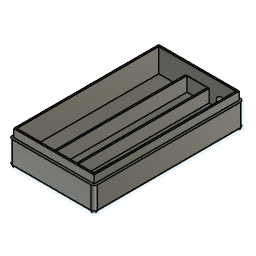
Controller_Left_Top v7 (Autodesk Fusion 360 design; units mm, degrees)
Autodesk Fusion 360 part; units mm, degrees
sketch "Sketch1" plane through (0, 0, 0) normal (0, 0, 1) x (1, 0, 0)
  line L0 (-27, -47.5) -> (27, -47.5)
  line L1 (27, -47.5) -> (27, 47.5)
  line L2 (27, 47.5) -> (-27, 47.5)
  line L3 (-27, 47.5) -> (-27, -47.5)
  line L4 (-27, -47.5) -> (27, 47.5) construction
  line L5 (27, -47.5) -> (-27, 47.5) construction
  dimension "d1" = 95
  dimension "d2" = 54
  constraint horizontal L0
  constraint perpendicular L0 L1
  constraint parallel L0 L2
  constraint parallel L1 L3
  constraint coincident L4 origin
  constraint coincident L5 origin
  measures "d1" distance of L0 L2
  measures "d2" distance of L1 L3
extrude "Extrude1" add sketch "Sketch1" along normal blind 11
sketch "Sketch2" plane through (0, 0, 11) normal (0, 0, 1) x (-1, 0, 0)
  line L0 (27, -47.5) -> (27, 47.5)
  line L1 (27, 47.5) -> (-27, 47.5)
  line L2 (-27, 47.5) -> (-27, -47.5)
  line L3 (-27, -47.5) -> (27, -47.5)
  line L4 (24.5, -45) -> (-24.5, -45)
  line L5 (-24.5, -45) -> (-24.5, 45)
  line L6 (-24.5, 45) -> (24.5, 45)
  line L7 (24.5, 45) -> (24.5, -45)
  line L8 (24.5, -45) -> (-24.5, 45) construction
  line L9 (-24.5, -45) -> (24.5, 45) construction
  dimension "d5" = 2.5
  dimension "d6" = 2.5
  dimension "d7" = 2.5
  dimension "d8" = 90
  constraint horizontal L4
  constraint perpendicular L4 L5
  constraint parallel L4 L6
  constraint parallel L5 L7
  constraint coincident L8 origin
  constraint coincident L9 origin
  measures "d5" distance of L3 L4
  measures "d6" distance of L1 L6
  measures "d7" distance of L2 L5
  measures "d8" distance of L4 L6
extrude "Extrude2" add sketch "Sketch2" along normal blind 5
extrude "Extrude3" cut 1 faces at (-8.1667, -15, 11) along direction (0, 0, -1) blind 5
sketch "Sketch3" plane through (0, 0, 6) normal (0, 0, 1) x (-1, 0, 0)
  line L0 (-24.5, 45) -> (-24.5, -45)
  line L1 (-24.5, -45) -> (24.5, -45)
  line L2 (24.5, -45) -> (24.5, 45)
  line L3 (24.5, 45) -> (-24.5, 45)
  line L4 (7.5, 45) -> (-7.5, 45)
  line L5 (-7.5, 45) -> (-7.5, -45)
  line L6 (-7.5, -45) -> (7.5, -45)
  line L7 (7.5, -45) -> (7.5, 45)
  line L8 (7.5, 45) -> (-7.5, -45) construction
  line L9 (-7.5, 45) -> (7.5, -45) construction
  dimension "d13" = 90
  dimension "d14" = 15
  constraint horizontal L4
  constraint perpendicular L4 L5
  constraint parallel L4 L6
  constraint parallel L5 L7
  constraint coincident L8 origin
  constraint coincident L9 origin
  measures "d13" distance of L4 L6
  measures "d14" distance of L5 L7
extrude "Extrude4" add sketch "Sketch3" along normal blind 8 contours L1 L3 L4 L5 L6 L7
sketch "Sketch4" plane through (0, 0, 14) normal (0, 0, 1) x (-1, 0, 0)
  line L0 (7.5, -45) -> (7.5, 45)
  line L1 (7.5, 45) -> (-7.5, 45)
  line L2 (-7.5, 45) -> (-7.5, -45)
  line L3 (-7.5, -45) -> (7.5, -45)
  line L4 (-6.5, 44.9) -> (6.5, 44.9)
  line L5 (6.5, 44.9) -> (6.5, -44.9)
  line L6 (6.5, -44.9) -> (-6.5, -44.9)
  line L7 (-6.5, -44.9) -> (-6.5, 44.9)
  line L8 (-6.5, 44.9) -> (6.5, -44.9) construction
  line L9 (6.5, 44.9) -> (-6.5, -44.9) construction
  dimension "d18" = 0.1
  dimension "d68" = 13
  constraint horizontal L4
  constraint perpendicular L4 L5
  constraint parallel L4 L6
  constraint parallel L5 L7
  constraint coincident L8 origin
  constraint coincident L9 origin
  measures "d18" distance of L3 L6
  measures "d68" distance of L5 L7
extrude "Extrude5" cut sketch "Sketch4" against normal blind 9 contours L4 L5 L6 L7
sketch "Sketch5" plane through (0, 0, 5) normal (0, 0, 1) x (-1, 0, 0)
  line L0 (-6.5, -44.9) -> (6.5, -44.9)
  line L1 (6.5, -44.9) -> (6.5, 44.9)
  line L2 (6.5, 44.9) -> (-6.5, 44.9)
  line L3 (-6.5, 44.9) -> (-6.5, -44.9)
  line L4 (-1.5, 36.5) -> (1.5, 36.5)
  line L5 (1.5, 36.5) -> (1.5, -36.5)
  line L6 (1.5, -36.5) -> (-1.5, -36.5)
  line L7 (-1.5, -36.5) -> (-1.5, 36.5)
  line L8 (-1.5, 36.5) -> (1.5, -36.5) construction
  line L9 (1.5, 36.5) -> (-1.5, -36.5) construction
  dimension "d21" = 3
  dimension "d22" = 73
  constraint horizontal L4
  constraint perpendicular L4 L5
  constraint parallel L4 L6
  constraint parallel L5 L7
  constraint coincident L8 origin
  constraint coincident L9 origin
  measures "d21" horizontal distance of L4.start L5.end
  measures "d22" distance of L4 L6
extrude "Extrude6" cut sketch "Sketch5" against normal blind 5 contours L4 L5 L6 L7
sketch "Sketch6" plane through (0, 0, 16) normal (0, 0, 1) x (-1, 0, 0)
  line L0 (-24.5, 45) -> (24.5, 45)
  line L1 (24.5, 45) -> (24.5, -45)
  line L2 (24.5, -45) -> (-24.5, -45)
  line L3 (-24.5, -45) -> (-24.5, 45)
  line L4 (-27, -47.5) -> (27, -47.5)
  line L5 (27, -47.5) -> (27, 47.5)
  line L6 (27, 47.5) -> (-27, 47.5)
  line L7 (-27, 47.5) -> (-27, -47.5)
  line L8 (-25.5, -46) -> (25.5, -46)
  line L9 (25.5, -46) -> (25.5, 46)
  line L10 (25.5, 46) -> (-25.5, 46)
  line L11 (-25.5, 46) -> (-25.5, -46)
  line L12 (-25.5, -46) -> (25.5, 46) construction
  line L13 (25.5, -46) -> (-25.5, 46) construction
  dimension "d25" = 1.5
  dimension "d26" = 1.5
  constraint horizontal L8
  constraint perpendicular L8 L9
  constraint parallel L8 L10
  constraint parallel L9 L11
  constraint coincident L12 origin
  constraint coincident L13 origin
  measures "d25" distance of L5 L9
  measures "d26" distance of L6 L10
extrude "Extrude7" add sketch "Sketch6" along normal blind 5 contours L8 L9 L10 L11
sketch "Sketch7" plane through (0, 47.5, 0) normal (0, 1, 0) x (-1, 0, 0)
  line L0 (-27, 0) -> (27, 0)
  line L1 (27, 0) -> (27, 16)
  line L2 (27, 16) -> (-27, 16)
  line L3 (-27, 16) -> (-27, 0)
  circle A0 centre (14.9884, 9.9657) radius 5
  dimension "d29" = 10
  measures "d29" diameter of A0
extrude "Extrude8" add sketch "Sketch7" along normal blind 2 contours A0
fillet "Fillet1" radius 1 1 edges at (-10.3267, 49.5, 8.1576)
sketch "Sketch8" plane through (0, 49.5, 0) normal (0, 1, 0) x (-1, 0, 0)
  circle A0 centre (14.9884, 9.9657) radius 4
sketch "Sketch9" plane through (0, 49.5, 0) normal (0, 1, 0) x (-1, 0, 0)
  circle A0 centre (14.9884, 9.9657) radius 3
  point P0 (14.9884, 9.9657)
  dimension "d34" = 6
  constraint coincident P0 A0.centre
  measures "d34" diameter of A0
extrude "Extrude9" cut sketch "Sketch9" against normal blind 5
sketch "Sketch10" plane through (0, 0, 0) normal (1, 0, 0) x (0, 1, 0)
sketch "Sketch11" plane through (0, 47.5, 0) normal (0, 1, 0) x (-1, 0, 0)
  circle A0 centre (14.9884, 9.9657) radius 5
  line L0 (-27, 0) -> (27, 0)
  line L1 (27, 0) -> (27, 16)
  line L2 (27, 16) -> (-27, 16)
  line L3 (-27, 16) -> (-27, 0)
pattern_linear "R-Pattern1" count 1 spacing 0 along (0, 1, 0) count 2 spacing 30 along (1, 0, 0) of "Extrude8", "Fillet1"
sketch "Sketch12" plane through (0, 49.5, 0) normal (0, 1, 0) x (-1, 0, 0)
  circle A0 centre (-15.0116, 9.9657) radius 4
  dimension "d69" = 8
  measures "d69" diameter of A0
extrude "Extrude10" cut sketch "Sketch12" against normal blind 5
extrude "Extrude11" add sketch "Sketch8" against normal blind 4.5
delete_face "DeleteFace1" 1 faces at (-19.3312, 48.8271, 7.6007)
delete_face "DeleteFace2" 1 faces at (-19.9635, 48.8333, 10.4635)
sketch "Sketch13" plane through (0, 0, 0) normal (0, 0, -1) x (1, 0, 0)
  line L0 (-1.5, -36.5) -> (-1.5, 36.5)
  line L1 (-1.5, 36.5) -> (1.5, 36.5)
  line L2 (1.5, 36.5) -> (1.5, -36.5)
  line L3 (1.5, -36.5) -> (-1.5, -36.5)
  line L4 (-27, 47.5) -> (-27, -47.5)
  line L5 (-27, -47.5) -> (27, -47.5)
  line L6 (27, -47.5) -> (27, 47.5)
  line L7 (27, 47.5) -> (-27, 47.5)
sketch "Sketch14" plane through (0, 0, 6) normal (0, 0, 1) x (-1, 0, 0)
  line L0 (-7.5, -45) -> (-7.5, 45)
  line L1 (-7.5, 45) -> (-24.5, 45)
  line L2 (-24.5, 45) -> (-24.5, -45)
  line L3 (-14.4887, -45) -> (-7.5, -45)
  line L4 (-9.3113, -19.1689) -> (-21.3113, -19.1689)
  line L5 (-21.3113, -19.1689) -> (-21.3113, -31.1689)
  line L6 (-21.3113, -31.1689) -> (-9.3113, -31.1689)
  line L7 (-9.3113, -31.1689) -> (-9.3113, -19.1689)
  line L8 (-9.3113, -19.1689) -> (-21.3113, -31.1689) construction
  line L9 (-21.3113, -19.1689) -> (-9.3113, -31.1689) construction
  line L10 (-15.5345, -45) -> (-15.5345, -44.5)
  line L11 (-15.5345, -44.5) -> (-14.4887, -44.5)
  line L12 (-14.4887, -44.5) -> (-14.4887, -45)
  line L13 (-24.5, -45) -> (-15.5345, -45)
  point P0 (-15.3113, -25.1689)
  dimension "d45" = 12
  dimension "d46" = 12
  constraint horizontal L4
  constraint perpendicular L4 L5
  constraint parallel L4 L6
  constraint parallel L5 L7
  constraint coincident L8 P0
  constraint coincident L9 P0
  measures "d45" distance of L4 L6
  measures "d46" distance of L5 L7
extrude "Extrude12" cut sketch "Sketch14" against normal blind 4 contours L4 L5 L6 L7
sketch "Sketch15" plane through (0, 0, 2) normal (0, 0, 1) x (-1, 0, 0)
  line L0 (-9.3113, -31.1689) -> (-9.3113, -19.1689)
  line L1 (-9.3113, -19.1689) -> (-21.3113, -19.1689)
  line L2 (-21.3113, -19.1689) -> (-21.3113, -31.1689)
  line L3 (-21.3113, -31.1689) -> (-9.3113, -31.1689)
  circle A0 centre (-15.3113, -25.1689) radius 5.5
  dimension "d49" = 11
  measures "d49" diameter of A0
extrude "Extrude13" cut sketch "Sketch15" against normal blind 10 contours A0
fillet "Fillet2" radius 2 4 edges at (27, -47.5, 8) (-27, -47.5, 8) (27, 47.5, 8) (-27, 47.5, 8)
fillet "Fillet3" radius 2 8 edges at (0, 47.5, 0) (-26.4142, 46.9142, 0) (-27, 0, 0) (-26.4142, -46.9142, 0) (0, -47.5, 0) (26.4142, -46.9142, 0) (27, 0, 0) (26.4142, 46.9142, 0)
pattern_linear "R-Pattern2" count 1 spacing 0 along (-1, 0, 0) count 2 spacing 50 along (0, -1, 0) of "Extrude12"
extrude "Extrude14" add 1 faces at (19.7983, 29.8493, 2) along direction (0, 0, 1) blind 4
sketch "Sketch16" plane through (0, 0, 6) normal (0, 0, 1) x (-1, 0, 0)
  circle A0 centre (-15.3113, -25.1689) radius 5.5
  line L0 (-21.3113, 30.8311) -> (-9.3113, 30.8311)
  line L1 (-9.3113, 30.8311) -> (-9.3113, 18.8311)
  line L2 (-9.3113, 18.8311) -> (-21.3113, 18.8311)
  line L3 (-21.3113, 18.8311) -> (-21.3113, 30.8311)
  line L4 (-7.5, -45) -> (-7.5, 45)
  line L5 (-7.5, 45) -> (-24.5, 45)
  line L6 (-24.5, 45) -> (-24.5, -45)
  line L7 (-14.4887, -45) -> (-7.5, -45)
  line L8 (-9.4631, -30.7737) -> (-21.1595, -30.7737)
  line L9 (-21.1595, -30.7737) -> (-21.1595, -19.5641)
  line L10 (-21.1595, -19.5641) -> (-9.4631, -19.5641)
  line L11 (-9.4631, -19.5641) -> (-9.4631, -30.7737)
  line L12 (-9.4631, -30.7737) -> (-21.1595, -19.5641) construction
  line L13 (-21.1595, -30.7737) -> (-9.4631, -19.5641) construction
  line L14 (-15.5345, -45) -> (-15.5345, -44.5)
  line L15 (-15.5345, -44.5) -> (-14.4887, -44.5)
  line L16 (-14.4887, -44.5) -> (-14.4887, -45)
  line L17 (-24.5, -45) -> (-15.5345, -45)
  point P0 (-15.3113, -25.1689)
  constraint horizontal L8
  constraint perpendicular L8 L9
  constraint parallel L8 L10
  constraint parallel L9 L11
  constraint coincident L12 P0
  constraint coincident L13 P0
  constraint coincident P0 A0.centre
extrude "Extrude15" add sketch "Sketch16" against normal blind 6 contours A0
sketch "Sketch17" plane through (0, 0, 2) normal (0, 0, 1) x (-1, 0, 0)
  line L0 (-9.3113, 18.8311) -> (-9.3113, 30.8311)
  line L1 (-9.3113, 30.8311) -> (-21.3113, 30.8311)
  line L2 (-21.3113, 30.8311) -> (-21.3113, 18.8311)
  line L3 (-21.3113, 18.8311) -> (-9.3113, 18.8311)
  circle A0 centre (-15.3113, 25.0362) radius 6
  dimension "d64" = 12
  dimension "d65" = 6
  measures "d64" diameter of A0
  measures "d65" distance of L0 A0.centre
extrude "Extrude16" cut sketch "Sketch17" against normal blind 6 contours L1 A0 picked at (-14.4604, 26.2072)
sketch "Sketch18" plane through (0, 49.5, 0) normal (0, 1, 0) x (-1, 0, 0)
extrude "Extrude17" add sketch "Sketch12" against normal blind 4.5
sketch "Sketch19" plane through (0, 49.5, 0) normal (0, 1, 0) x (-1, 0, 0)
  circle A0 centre (-15.0116, 9.9657) radius 4
  circle A1 centre (-15.0116, 9.9657) radius 3
  dimension "d72" = 6
  constraint concentric A0 A1
  measures "d72" diameter of A1
extrude "Extrude18" cut sketch "Sketch19" against normal blind 6 contours A1
